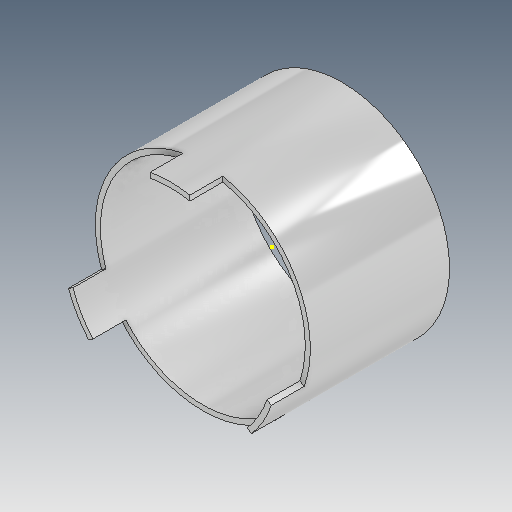
# Autodesk Inventor part: Inner part of servo motor
Saved by Autodesk Inventor 2020.3 (Build 243373010, 373A)
## iProperties
Created: 2021-04-08
Part Number: Inner part of servo motor
Material: Aluminum 6061-AHC
Document SubType Name: Modeling
Designer: marti
Density: 2.7 g/cm^3
Appearance: Aluminum - Dark
Mass: 10.0904 g
Surface Area: 77.7469 cm^2
Volume: 3.73719 cm^3
Author: marti
Autodesk Inventor part; units mm, degrees
ref_plane "YZ Plane" through (0, 0, 0) normal (1, 0, 0) x (0, 1, 0)
ref_plane "XZ Plane" through (0, 0, 0) normal (0, 1, 0) x (-1, 0, 0)
sketch "Sketch1" plane through (0, 0, 0) normal (0, 0, 1) x (1, 0, 0)
  circle A0 centre (0, 0) radius 21.2375
  circle A1 centre (0, 0) radius 20.2375
  dimension "d0" = 42.475
  dimension "d1" = 1
  constraints: 2 centre point, 1 coincident
  measures "d0" diameter of A0
  measures "d1" radial gap between concentric circles of A0 A1
extrude "Extrusion1" add sketch "Sketch1" along normal mid plane 27.5
sketch "Sketch2" plane through (0, 0, 13.75) normal (0, 0, 1) x (1, 0, 0)
  circle A0 centre (0, 0) radius 21.2375 projected
  circle A1 centre (0, 0) radius 20.2375 projected
  line L0 (-3.925, 20.8717) -> (-3.925, 19.8532)
  line L1 (3.925, 20.8717) -> (3.925, 19.8532)
  point P0 (0, 13.5869)
  dimension "d4" = 7.85
  constraints: 4 end point, 4 point on circle, 2 vertical, 1 vertical alignment
  measures "d4" distance between parallel lines of L0 L1
extrude "Extrusion2" add sketch "Sketch2" along normal blind 6.5 contours L1 A1 L0 A0 picked at (3.0552, 20.3065)
pattern_circular "Circular Pattern1" count 3 over 360 about axis through (0, 0, -10) along (0, 0, 1) of "Extrusion2"
sketch "Sketch3" plane through (0, 0, 0) normal (0, 0, 1) x (1, 0, 0)
  point P0 (0, 0)
ref_plane "Work Plane1" through (0, 0, 20.25) normal (0, 0, 1) x (1, 0, 0)
body "Solid1"
